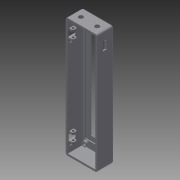
# Autodesk Inventor part: ESP_DISP_COVER
Saved by Autodesk Inventor 2015 (Build 190159000, 159)
## iProperties
Created: 2018-04-03
Part Number: ESP_DISP_COVER
Material: Типовые
Document SubType Name: Modeling
Designer: JOK
Density: 1 g/cm^3
Appearance: По умолчанию
Author: JOK
Autodesk Inventor part; units mm, degrees
ref_plane "YZ Plane" through (0, 0, 0) normal (1, 0, 0) x (0, 1, 0)
ref_plane "XZ Plane" through (0, 0, 0) normal (0, 1, 0) x (-1, 0, 0)
ref_plane "XY Plane" through (0, 0, 0) normal (0, 0, 1) x (1, 0, 0)
sketch "Эскиз1" plane through (0, 0, 0) normal (0, 1, 0) x (-1, 0, 0)
  line L0 (-20, 90) -> (20, 90)
  line L1 (20, 90) -> (20, -90)
  line L2 (20, -90) -> (-20, -90)
  line L3 (-20, -90) -> (-20, 90)
  line L4 (-20, 90) -> (20, -90) construction
  line L5 (20, 90) -> (-20, -90) construction
  line L6 (16, -86) -> (-16, -86)
  line L7 (-16, -86) -> (-16, 86)
  line L8 (-16, 86) -> (16, 86)
  line L9 (16, 86) -> (16, -86)
  line L10 (16, -86) -> (-16, 86) construction
  line L11 (-16, -86) -> (16, 86) construction
  line L12 (-11, 74) -> (11, 74)
  line L13 (11, 74) -> (11, -74)
  line L14 (11, -74) -> (-11, -74)
  line L15 (-11, -74) -> (-11, 74)
  line L16 (-11, 74) -> (11, -74) construction
  line L17 (11, 74) -> (-11, -74) construction
  circle A0 centre (16, 86) radius 1.6
  line L18 (17.7, 80.7) -> (-17.7, 80.7)
  line L19 (-17.7, 80.7) -> (-17.7, -80.7)
  line L20 (-17.7, -80.7) -> (17.7, -80.7)
  line L21 (17.7, -80.7) -> (17.7, 80.7)
  line L22 (17.7, 80.7) -> (-17.7, -80.7) construction
  line L23 (-17.7, 80.7) -> (17.7, -80.7) construction
  line L24 (-8.89, -88.5) -> (8.89, -88.5)
  line L25 (8.89, -88.5) -> (8.89, -83.5)
  line L26 (8.89, -83.5) -> (-8.89, -83.5)
  line L27 (-8.89, -83.5) -> (-8.89, -88.5)
  line L28 (-8.89, -88.5) -> (8.89, -83.5) construction
  line L29 (8.89, -88.5) -> (-8.89, -83.5) construction
  point P0 (0, 0)
  point P1 (0, -86)
  dimension "d0" = 40
  dimension "d1" = 180
  dimension "d2" = 32
  dimension "d3" = 172
  dimension "d4" = 22
  dimension "d5" = 148
  dimension "d6" = 3.2
  dimension "d7" = 35.4
  dimension "d8" = 161.4
  dimension "d21" = 17.78
  dimension "d22" = 5
  constraints: 60 end point, 11 midpoint, 10 parallel, 5 coincident, 5 horizontal, 5 perpendicular, 1 centre point
  measures "d0" distance of L1.end L2.end
  measures "d1" distance of L0.end L1.end
  measures "d2" distance of L7.end L8.end
  measures "d3" distance of L6.end L7.end
  measures "d4" distance of L13.end L14.end
  measures "d5" distance of L12.end L13.end
  measures "d6" diameter of A0
  measures "d7" distance of L20.end L19.end
  measures "d8" distance of L19.end L18.end
  measures "d21" distance of L26.end L25.end
  measures "d22" distance of L25.end L24.end
sketch "Эскиз2" plane through (0, 0, 0) normal (0, 1, 0) x (-1, 0, 0)
  line L0 (25, 95) -> (-25, 95)
  line L1 (-25, 95) -> (-25, -95)
  line L2 (-25, -95) -> (25, -95)
  line L3 (25, -95) -> (25, 95)
  line L4 (25, 95) -> (-25, -95) construction
  line L5 (-25, 95) -> (25, -95) construction
  line L6 (11, -74) -> (-11, -74)
  line L7 (-11, -74) -> (-11, 74)
  line L8 (-11, 74) -> (11, 74)
  line L9 (11, 74) -> (11, -74)
  line L10 (11, -74) -> (-11, 74) construction
  line L11 (-11, -74) -> (11, 74) construction
  point P0 (0, 0)
  dimension "d9" = 50
  dimension "d10" = 190
  constraints: 24 end point, 4 midpoint, 4 parallel, 2 horizontal, 2 perpendicular
  measures "d9" distance of L2.end L1.end
  measures "d10" distance of L1.end L0.end
extrude "Выдавливание1" add sketch "Эскиз2" along normal blind 3
sketch "Эскиз3" plane through (0, 0, 0) normal (0, -1, 0) x (1, 0, 0)
  line L0 (-25, 95) -> (25, 95) projected
  line L1 (-25, -95) -> (-25, 95) projected
  line L2 (25, -95) -> (-25, -95) projected
  line L3 (25, 95) -> (25, -95) projected
  line L4 (-22, 92) -> (22, 92)
  line L5 (22, 92) -> (22, -92)
  line L6 (22, -92) -> (-22, -92)
  line L7 (-22, -92) -> (-22, 92)
  line L8 (-22, 92) -> (22, -92) construction
  line L9 (22, 92) -> (-22, -92) construction
  point P0 (0, 0)
  dimension "d13" = 44
  dimension "d14" = 184
  constraints: 12 end point, 2 midpoint, 2 parallel, 1 horizontal, 1 perpendicular
  measures "d13" distance of L5.end L6.end
  measures "d14" distance of L4.end L5.end
extrude "Выдавливание2" add sketch "Эскиз3" along normal blind 24
sketch "Эскиз4" plane through (0, 0, 0) normal (0, -1, 0) x (1, 0, 0)
  circle A0 centre (-16, -86) radius 4
  circle A1 centre (16, -86) radius 4
  circle A2 centre (16, 86) radius 4
  circle A3 centre (-16, 86) radius 4
  point P0 (0, 0)
  dimension "d17" = 8
  dimension "d18" = 8
  dimension "d19" = 8
  dimension "d20" = 8
  constraints: 4 centre point
  measures "d17" diameter of A0
  measures "d18" diameter of A1
  measures "d19" diameter of A2
  measures "d20" diameter of A3
extrude "Выдавливание3" add sketch "Эскиз4" along normal blind 4
sketch "Эскиз5" plane through (22, 0, 92) normal (0, 0, -1) x (-1, 0, 0)
  line L0 (0, 0) -> (44, 0) projected
  line L1 (0, 0) -> (0, -24) projected
  line L2 (44, -24) -> (0, -24) projected
  line L3 (44, 0) -> (44, -24) projected
  line L4 (0, -12) -> (44, -12)
  line L5 (22, -24) -> (22, 0)
  line L6 (22, -12) -> (35, -12)
  circle A0 centre (35, -12) radius 3.5
  line L7 (44, -12) -> (0, -12)
  circle A1 centre (9, -12) radius 3.5
  dimension "d25" = 13
  dimension "d26" = 7
  constraints: 8 end point, 4 midpoint, 3 symmetric about line, 2 centre point, 1 coincident, 1 perpendicular, 1 point on line, 1 other
  measures "d25" distance of L6.start L6.end
  measures "d26" diameter of A0
extrude "Выдавливание4" cut sketch "Эскиз5" against normal blind 5.2 contours A1 L4 | L4 A1 | A0 L4 | L4 A0
sketch "Эскиз6" plane through (22, 0, 92) normal (0, 0, -1) x (-1, 0, 0)
  circle A0 centre (9, -12) radius 3.5 projected
  circle A1 centre (35, -12) radius 3.5 projected
  circle A2 centre (35, -12) radius 5.5
  circle A3 centre (9, -12) radius 5.5
  point P0 (22, 0)
  dimension "d29" = 11
  dimension "d30" = 11
  constraints: 2 centre point, 2 coincident
  measures "d29" diameter of A2
  measures "d30" diameter of A3
extrude "Выдавливание5" cut sketch "Эскиз6" against normal blind 1
fillet "Сопряжение1" radius 1 4 edges at (16.5, -12, 93) (-9.5, -12, 93) (-7.5, -12, 92) (18.5, -12, 92)
sketch "Эскиз7" plane through (-16, -4, 86) normal (0, -1, 0) x (1, 0, 0)
  circle A0 centre (0, 0) radius 4 projected
  circle A1 centre (0, 0) radius 2.5
  point P0 (16, -86)
  dimension "d34" = 5
  constraints: 1 centre point, 1 coincident
  measures "d34" diameter of A1
extrude "Выдавливание6" cut sketch "Эскиз7" against normal blind 4 contours A1
sketch "Эскиз8" plane through (16, -4, 86) normal (0, -1, 0) x (1, 0, 0)
  circle A0 centre (0, 0) radius 4 projected
  circle A1 centre (0, 0) radius 2.5
  circle A2 centre (0, -172) radius 2.5
  circle A3 centre (-32, -172) radius 2.5
  point P0 (-16, -86)
  dimension "d37" = 5
  dimension "d38" = 5
  dimension "d39" = 5
  constraints: 3 centre point, 1 coincident
  measures "d37" diameter of A1
  measures "d38" diameter of A2
  measures "d39" diameter of A3
extrude "Выдавливание7" cut sketch "Эскиз8" against normal blind 4 contours A1 | A2 | A3
sketch "Эскиз9" plane through (0, 0, 0) normal (0, -1, 0) x (1, 0, 0)
  line L0 (11, 74) -> (11, -74) projected
  line L1 (11, -74) -> (-11, -74) projected
  line L2 (-11, -74) -> (-11, 74) projected
  line L3 (-11, 74) -> (11, 74) projected
  line L4 (-18.5, 81.5) -> (18.5, 81.5)
  line L5 (18.5, 81.5) -> (18.5, -81.5)
  line L6 (18.5, -81.5) -> (-18.5, -81.5)
  line L7 (-18.5, -81.5) -> (-18.5, 81.5)
  line L8 (-18.5, 81.5) -> (18.5, -81.5) construction
  line L9 (18.5, 81.5) -> (-18.5, -81.5) construction
  point P0 (0, 0)
  dimension "d42" = 37
  dimension "d43" = 163
  constraints: 12 end point, 2 midpoint, 2 parallel, 1 horizontal, 1 perpendicular
  measures "d42" distance of L5.end L6.end
  measures "d43" distance of L4.end L5.end
extrude "Выдавливание8" cut sketch "Эскиз9" against normal blind 1.5
sketch "Эскиз10" plane through (22, 0, -92) normal (-1, 0, 0) x (0, 0, 1)
  line L0 (184, -24) -> (0, -24) projected
  line L1 (184, 0) -> (184, -24) projected
  line L2 (184, -24) -> (167, -24)
  line L3 (167, -24) -> (167, 0)
  line L4 (173.5, 0) -> (10.5, 0) projected
  line L5 (167, -24) -> (191, -24) construction
  line L6 (167, -12) -> (184, -12)
  line L7 (160, -9) -> (174, -9)
  line L8 (174, -9) -> (174, -15)
  line L9 (174, -15) -> (160, -15)
  line L10 (160, -15) -> (160, -9)
  line L11 (160, -9) -> (174, -15) construction
  line L12 (174, -9) -> (160, -15) construction
  point P0 (92, 0)
  dimension "d46" = 90
  dimension "d47" = 14
  dimension "d48" = 6
  constraints: 20 end point, 4 midpoint, 2 horizontal, 2 parallel, 2 perpendicular, 2 point on line
  measures "d46" angle of L5 L3
  measures "d47" distance of L8.end L9.end
  measures "d48" distance of L7.end L8.end
extrude "Выдавливание9" cut sketch "Эскиз10" against normal blind 3 contours L9 L10 L7 L3 | L3 L6 L8 L9 | L6 L3 L7 L8
sketch "Эскиз11" plane through (22, 0, -92) normal (-1, 0, 0) x (0, 0, 1)
  line L0 (160, -15) -> (160, -9) projected
  line L1 (160, -9) -> (174, -9) projected
  line L2 (174, -9) -> (174, -15) projected
  line L3 (174, -15) -> (160, -15) projected
  line L4 (158.5, -7.5) -> (175.5, -7.5)
  line L5 (175.5, -7.5) -> (175.5, -16.5)
  line L6 (175.5, -16.5) -> (158.5, -16.5)
  line L7 (158.5, -16.5) -> (158.5, -7.5)
  line L8 (158.5, -7.5) -> (175.5, -16.5) construction
  line L9 (175.5, -7.5) -> (158.5, -16.5) construction
  point P0 (92, 0)
  point P1 (167, -12)
  dimension "d51" = 17
  dimension "d52" = 9
  constraints: 12 end point, 2 midpoint, 2 parallel, 1 horizontal, 1 perpendicular
  measures "d51" distance of L5.end L6.end
  measures "d52" distance of L4.end L5.end
extrude "Выдавливание10" cut sketch "Эскиз11" against normal blind 1
fillet "Сопряжение2" radius 0.5 8 edges at (23, -12, 82) (23, -9, 75) (23, -15, 75) (23, -12, 68) (22, -12, 83.5) (22, -16.5, 75) (22, -7.5, 75) (22, -12, 66.5)
sketch "Эскиз12" plane through (-25, 3, -95) normal (-1, 0, 0) x (0, 0, 1)
  line L0 (190, 0) -> (190, -27) projected
  line L1 (190, -27) -> (0, -27) projected
  line L2 (190, -13.5) -> (0, -13.5)
  line L3 (0, -27) -> (0, 0) projected
  line L4 (190, -13.5) -> (166, -13.5)
  line L5 (0, -13.5) -> (24, -13.5)
  line L6 (0, -13.5) -> (24, -13.5) construction
  line L7 (24, -13.5) -> (24, -27)
  line L8 (29, -16.75) -> (19, -16.75)
  line L9 (19, -16.75) -> (19, -23.75)
  line L10 (19, -23.75) -> (29, -23.75)
  line L11 (29, -23.75) -> (29, -16.75)
  line L12 (29, -16.75) -> (19, -23.75) construction
  line L13 (19, -16.75) -> (29, -23.75) construction
  line L14 (24, -20.25) -> (190, -20.25)
  line L15 (190, -13.5) -> (166, -13.5)
  line L16 (171, -16.75) -> (161, -16.75)
  line L17 (161, -16.75) -> (161, -23.75)
  line L18 (161, -23.75) -> (171, -23.75)
  line L19 (171, -23.75) -> (171, -16.75)
  line L20 (171, -16.75) -> (161, -23.75) construction
  line L21 (161, -16.75) -> (171, -23.75) construction
  point P0 (95, -3)
  point P1 (166, -20.25)
  dimension "d56" = 24
  dimension "d57" = 0
  dimension "d58" = 10
  dimension "d59" = 7
  dimension "d62" = 24
  dimension "d63" = 10
  dimension "d64" = 7
  constraints: 38 end point, 7 midpoint, 4 horizontal, 4 parallel, 4 point on line, 3 collinear, 3 perpendicular
  measures "d56" distance of L2.end L5.end
  measures "d57" distance between parallel lines of L5 L6
  measures "d58" distance of L10.end L9.end
  measures "d59" distance of L9.end L8.end
  measures "d62" distance of L2.start L4.end
  measures "d63" distance of L18.end L17.end
  measures "d64" distance of L17.end L16.end
extrude "Выдавливание11" cut sketch "Эскиз12" against normal blind 4 contours L19 L18 L17 L14 | L14 L17 L16 L19 | L8 L11 L14 L7 | L7 L10 L9 L8 | L7 L14 L11 L10
sketch "Эскиз13" plane through (-22, 0, 92) normal (1, 0, 0) x (0, 0, -1)
  line L0 (26, -13.75) -> (29, -13.75)
  line L1 (29, -13.75) -> (29, -20.75)
  line L2 (29, -20.75) -> (26, -20.75)
  line L3 (26, -20.75) -> (26, -13.75)
  line L4 (16, -20.75) -> (13, -20.75)
  line L5 (13, -20.75) -> (13, -13.75)
  line L6 (13, -13.75) -> (16, -13.75)
  line L7 (16, -13.75) -> (16, -20.75)
  line L8 (158, -20.75) -> (155, -20.75)
  line L9 (155, -20.75) -> (155, -13.75)
  line L10 (155, -13.75) -> (158, -13.75)
  line L11 (158, -13.75) -> (158, -20.75)
  line L12 (168, -20.75) -> (171, -20.75)
  line L13 (171, -20.75) -> (171, -13.75)
  line L14 (171, -13.75) -> (168, -13.75)
  line L15 (168, -13.75) -> (168, -20.75)
  line L16 (155, -13.75) -> (151, -13.75)
  line L17 (151, -13.75) -> (151, -20.75)
  line L18 (151, -20.75) -> (155, -20.75)
  line L19 (155, -20.75) -> (155, -13.75)
  line L20 (171, -20.75) -> (175, -20.75)
  line L21 (175, -20.75) -> (175, -13.75)
  line L22 (175, -13.75) -> (171, -13.75)
  line L23 (171, -13.75) -> (171, -20.75)
  line L24 (29, -20.75) -> (33, -20.75)
  line L25 (33, -20.75) -> (33, -13.75)
  line L26 (33, -13.75) -> (29, -13.75)
  line L27 (29, -13.75) -> (29, -20.75)
  line L28 (13, -20.75) -> (9, -20.75)
  line L29 (9, -20.75) -> (9, -13.75)
  line L30 (9, -13.75) -> (13, -13.75)
  line L31 (13, -13.75) -> (13, -20.75)
  point P0 (92, 0)
  constraints: 64 end point, 16 parallel, 8 horizontal, 8 perpendicular, 5 point on line
extrude "Выдавливание12" add sketch "Эскиз13" along normal blind 5 contours L0 L1 L2 L3 | L4 L5 L6 L7 | L8 L9 L10 L11 | L15 L14 L13 L12
extrude "Выдавливание13" cut sketch "Эскиз13" against normal blind 1 contours L26 L25 L24 L1 | L28 L29 L30 L5 | L18 L17 L16 L9 | L13 L22 L21 L20
fillet "Сопряжение3" radius 2 8 edges at (-17, -20.75, 64.5) (-17, -20.75, 77.5) (-17, -13.75, 77.5) (-17, -13.75, 64.5) (-17, -20.75, -64.5) (-17, -13.75, -64.5) (-17, -20.75, -77.5) (-17, -13.75, -77.5)
sketch "Эскиз14" plane through (-22, -20.75, -79) normal (0, 0, -1) x (-1, 0, 0)
  line L0 (-5, 2) -> (-5, 5) projected
  line L1 (0, 0) -> (-3, 0) projected
  line L2 (1, 0) -> (1, 7) projected
  line L3 (0, 7) -> (-3, 7) projected
  line L4 (1, 3.5) -> (-5, 3.5)
  line L5 (-5, 3.5) -> (-2, 3.5)
  line L6 (-2, 0) -> (-2, 7)
  line L7 (0, 7) -> (-3, 7) projected
  circle A0 centre (-2, 3.5) radius 1.75
  point P0 (-22, 20.75)
  dimension "d72" = 3.5
  constraints: 6 end point, 3 midpoint, 2 point on line, 1 centre point, 1 coincident, 1 perpendicular
  measures "d72" diameter of A0
extrude "Выдавливание14" cut sketch "Эскиз14" against normal blind 160
sketch "Эскиз15" plane through (22, 0, 92) normal (0, 0, -1) x (-1, 0, 0)
  line L0 (44, -24) -> (0, -24) projected
  line L1 (22, -24) -> (22, 0)
  line L2 (22, -21.25) -> (9.3, -21.25)
  line L3 (22, -21.25) -> (34.7, -21.25)
  line L4 (34.7, -21.25) -> (22, -21.25)
  line L5 (22, -21.25) -> (22, -6.01)
  circle A0 centre (9.3, -21.25) radius 0.6
  circle A1 centre (34.7, -21.25) radius 0.6
  circle A2 centre (22, -6.01) radius 0.6
  dimension "d75" = 12.7
  dimension "d76" = 12.7
  dimension "d77" = 15.24
  dimension "d78" = 1.2
  dimension "d79" = 1.2
  dimension "d80" = 1.2
  constraints: 10 end point, 3 centre point, 3 coincident, 1 collinear, 1 horizontal, 1 midpoint, 1 point on line, 1 vertical
  measures "d75" distance of L2.start L2.end
  measures "d76" distance of L2.start L3.end
  measures "d77" distance of L2.start L5.end
  measures "d78" diameter of A0
  measures "d79" diameter of A1
  measures "d80" diameter of A2
extrude "Выдавливание15" add sketch "Эскиз15" along normal blind 3
sketch "Эскиз16" plane through (22, 0, -92) normal (-1, 0, 0) x (0, 0, 1)
  line L0 (176, -17) -> (176, -7) projected
  line L1 (176, -12) -> (177, -12)
  line L2 (177, -12) -> (156.68, -12)
  line L3 (177, -18.7951) -> (156.68, -18.7951)
  line L4 (156.68, -18.7951) -> (156.68, -5.2049)
  line L5 (156.68, -5.2049) -> (177, -5.2049)
  line L6 (177, -5.2049) -> (177, -18.7951)
  line L7 (177, -18.7951) -> (156.68, -5.2049) construction
  line L8 (156.68, -18.7951) -> (177, -5.2049) construction
  circle A0 centre (156.68, -12) radius 0.6
  circle A1 centre (177, -12) radius 0.6
  circle A2 centre (166.84, -18.7951) radius 0.6
  circle A3 centre (166.84, -5.2049) radius 0.6
  point P0 (92, 0)
  point P1 (166.84, -12)
  dimension "d83" = 20.32
  dimension "d84" = 1.2
  dimension "d85" = 1.2
  dimension "d86" = 1.2
  dimension "d87" = 1.2
  constraints: 16 end point, 6 midpoint, 4 centre point, 2 coincident, 2 horizontal, 2 parallel, 1 perpendicular, 1 point on line
  measures "d83" distance of L1.end L2.end
  measures "d84" diameter of A0
  measures "d85" diameter of A1
  measures "d86" diameter of A2
  measures "d87" diameter of A3
extrude "Выдавливание16" add sketch "Эскиз16" along normal blind 3 contours A1 L6 L1 | L1 L6 A1 | A0 L4 L2 | L2 L4 A0 | L6 A1 | L4 A0 | A3 L5 | L5 A3 | A2 L3 | L3 A2
fillet "Сопряжение4" radius 3 8 edges at (-25, 3, 0) (-25, -10.5, -95) (-25, -10.5, 95) (0, 3, -95) (25, 3, 0) (0, 3, 95) (25, -10.5, -95) (25, -10.5, 95)
fillet "Сопряжение5" radius 1 4 edges at (-11, 3, 0) (0, 3, 74) (11, 3, 0) (0, 3, -74)
sketch "Эскиз17" plane through (-22, 0, 92) normal (1, 0, 0) x (0, 0, -1)
  line L0 (16, -13.75) -> (26, -13.75)
  line L1 (26, -13.75) -> (26, -11.75)
  line L2 (26, -11.75) -> (16, -11.75)
  line L3 (16, -11.75) -> (16, -13.75)
  line L4 (16, -20.75) -> (26, -20.75)
  line L5 (26, -20.75) -> (26, -22.25)
  line L6 (26, -22.25) -> (16, -22.25)
  line L7 (16, -22.25) -> (16, -20.75)
  line L8 (158, -20.75) -> (168, -20.75)
  line L9 (168, -20.75) -> (168, -22.25)
  line L10 (168, -22.25) -> (158, -22.25)
  line L11 (158, -22.25) -> (158, -20.75)
  line L12 (158, -13.75) -> (168, -13.75)
  line L13 (168, -13.75) -> (168, -11.75)
  line L14 (168, -11.75) -> (158, -11.75)
  line L15 (158, -11.75) -> (158, -13.75)
  point P0 (92, 0)
  dimension "d92" = 2
  dimension "d93" = 1.5
  dimension "d94" = 1.5
  dimension "d95" = 2
  constraints: 32 end point, 8 parallel, 4 horizontal, 4 perpendicular, 2 point on line
  measures "d92" distance of L1.end L0.end
  measures "d93" distance of L4.end L5.end
  measures "d94" distance of L8.end L9.end
  measures "d95" distance of L13.end L12.end
extrude "Выдавливание17" cut sketch "Эскиз17" against normal blind 10
chamfer "Фаска1" distance 3 angle 45 2 edges at (-25, -11.75, 71) (-25, -11.75, -71)
fillet "Сопряжение6" radius 1 2 edges at (-25, -22.25, 71) (-25, -22.25, -71)
